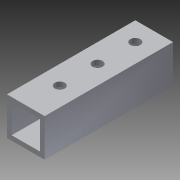
# Autodesk Inventor part: corner bumper mount
Saved by Autodesk Inventor 2014 SP1 (Build 180222100, 222)
## iProperties
Created: 2014-01-05
Part Number: corner bumper mount
Material: Aluminum 6061
Document SubType Name: Modeling
Designer: Arpan
Density: 2.71 g/cm^3
Appearance: Aluminum - Flat
Author: Arpan
Autodesk Inventor part; units mm, degrees
ref_plane "YZ Plane" through (0, 0, 0) normal (1, 0, 0) x (0, 1, 0)
ref_plane "XZ Plane" through (0, 0, 0) normal (0, 1, 0) x (-1, 0, 0)
ref_plane "XY Plane" through (0, 0, 0) normal (0, 0, 1) x (1, 0, 0)
sketch "Sketch1" plane through (0, 0, 0) normal (0, 0, 1) x (1, 0, 0)
  line L0 (0, 0) -> (-25.4, 0)
  line L1 (-25.4, 0) -> (-25.4, 25.4)
  line L2 (-25.4, 25.4) -> (0, 25.4)
  line L3 (0, 25.4) -> (0, 0)
  line L4 (-3.175, 22.225) -> (-22.225, 22.225)
  line L5 (-22.225, 22.225) -> (-22.225, 3.175)
  line L6 (-22.225, 3.175) -> (-3.175, 3.175)
  line L7 (-3.175, 3.175) -> (-3.175, 22.225)
  dimension "d0" = 25.4
  dimension "d1" = 25.4
  dimension "d2" = 3.175
  constraints: 16 end point, 4 parallel, 2 perpendicular, 1 horizontal, 3 other
  measures "d0" distance of L2.end L0.start
  measures "d1" distance of L0.start L0.end
  measures "d2" distance between parallel lines of L2 L4
extrude "Extrusion1" add sketch "Sketch1" along normal blind 86.36
sketch "Sketch2" plane through (-25.4, 25.4, 0) normal (0, 1, 0) x (1, 0, 0)
  line L0 (0, 0) -> (25.4, 0) projected
  line L1 (25.4, 0) -> (25.4, -86.36) projected
  line L2 (12.7, 0) -> (12.7, -12.7)
  circle A0 centre (12.7, -12.7) radius 3.3782
  dimension "d5" = 12.7
  dimension "d6" = 6.7564
  constraints: 2 end point, 1 centre point, 1 coincident, 1 midpoint, 1 parallel
  measures "d5" distance of L2.start L2.end
  measures "d6" diameter of A0
extrude "Extrusion2" cut sketch "Sketch2" against normal blind 86.36
pattern_linear "Rectangular Pattern1" count 3 spacing 25.4 along (0, 0, 1) of "Extrusion2"
body "Solid1"
